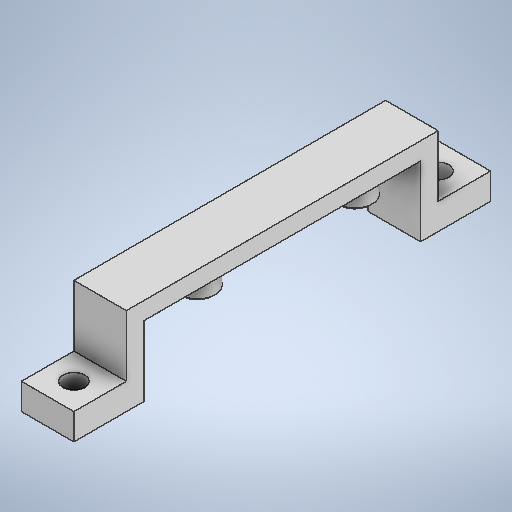
# Autodesk Inventor part: housing_xl320
Saved by Autodesk Inventor 2025 (Build 290162000, 162)
## iProperties
Created: 2025-10-20
Part Number: housing_xl320
Material: 一般
Document SubType Name: Modeling
Designer: sooo1
Density: 1 g/cm^3
Appearance: 既定
Author: sooo1
Autodesk Inventor part; units mm, degrees
ref_plane "YZ Plane" through (0, 0, 0) normal (1, 0, 0) x (0, 1, 0)
ref_plane "XZ Plane" through (0, 0, 0) normal (0, 1, 0) x (-1, 0, 0)
ref_plane "XY Plane" through (0, 0, 0) normal (0, 0, 1) x (1, 0, 0)
sketch "スケッチ1" plane through (0, 0, 0) normal (0, 1, 0) x (-1, 0, 0)
  line L0 (3, 26.15) -> (-3, 26.15)
  line L1 (-3, 26.15) -> (-3, -21.5)
  line L2 (-3, -21.5) -> (3, -21.5)
  line L3 (3, -21.5) -> (3, 26.15)
  line L4 (4.2, 0) -> (-4.2, 0) construction
  line L5 (4.2, 9) -> (-4.2, 9) construction
  line L6 (4.2, -9) -> (-4.2, -9) construction
  line L7 (0, -31.03) -> (0, 35.68) construction
  circle A0 centre (0, 9) radius 2
  circle A1 centre (0, -9) radius 2
  line L8 (0, 26.15) -> (0, -21.5) construction
  line L9 (3, 20.15) -> (-3, 20.15)
  line L10 (3, -15.5) -> (-3, -15.5)
  line L11 (3, 26.15) -> (-3, 20.15) construction
  line L12 (3, -15.5) -> (-3, -21.5) construction
  circle A2 centre (0, 23.15) radius 1.25
  circle A3 centre (0, -18.5) radius 1.25
  line L13 (-3, 18.15) -> (3, 18.15)
  line L14 (-3, -13.5) -> (3, -13.5)
  point P0 (0, 0)
  dimension "d0" = 6
  dimension "d1" = 9
  dimension "d2" = 9
  dimension "d3" = 4
  dimension "d4" = 12.5
  dimension "d5" = 17.15
  dimension "d6" = 6
  dimension "d7" = 6
  dimension "d8" = 2.5
  dimension "d11" = 4.5
  dimension "d12" = 9.15
  constraints: 26 end point, 10 point on line, 7 midpoint, 5 perpendicular, 4 centre point, 4 parallel, 2 equal radius, 1 collinear, 1 horizontal
  measures "d0" distance of L0.start L0.end
  measures "d1" distance between parallel lines of L4 L5
  measures "d2" distance between parallel lines of L4 L6
  measures "d3" diameter of A0
  measures "d4" distance between parallel lines of L6 L2
  measures "d5" distance between parallel lines of L5 L0
  measures "d6" distance between parallel lines of L2 L10
  measures "d7" distance between parallel lines of L0 L9
  measures "d8" diameter of A2
  measures "d11" distance from line of A1.centre L14
  measures "d12" distance from line of A0.centre L13
extrude "押し出し1" add sketch "スケッチ1" along normal blind 2 contours L3 L13 L1 L9 | L3 L14 L1 L13 | L3 L10 L1 L14 | A0 | A1
extrude "押し出し2" add sketch "スケッチ1" against normal blind 8 contours L3 L13 L1 L9 | L3 L10 L1 L14
extrude "押し出し3" add sketch "スケッチ1" along normal blind 3 from surface at -8 contours L3 L9 L1 L0 | L3 L2 L1 L10
extrude "押し出し4" add sketch "スケッチ1" against normal blind 2.8 contours A0 | A1
chamfer "面取り1" distance 0.3 angle 45 2 edges at (2, -2.8, 9) (2, -2.8, -9)
